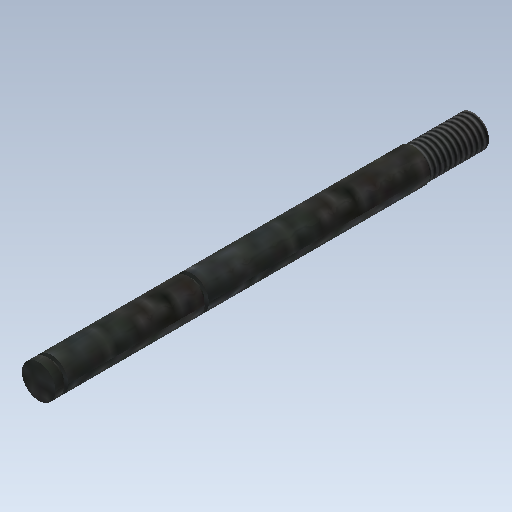
# Autodesk Inventor part: 500-104
Saved by Autodesk Inventor 2020 (Build 240168000, 168)
## iProperties
Created: 2015-04-18
Part Number: 500-104
Material: Steel
Document SubType Name: Modeling
Designer: Station9
Density: 7.85 g/cm^3
Appearance: Plate
Mass: 2.53931 g
Surface Area: 4.39374 cm^2
Volume: 0.323479 cm^3
Author: Station9
Autodesk Inventor part; units mm, degrees
ref_plane "YZ Plane" through (0, 0, 0) normal (1, 0, 0) x (0, 1, 0)
ref_plane "XZ Plane" through (0, 0, 0) normal (0, 1, 0) x (-1, 0, 0)
ref_plane "XY Plane" through (0, 0, 0) normal (0, 0, 1) x (1, 0, 0)
sketch "Sketch1" plane through (0, 0, 0) normal (0, 1, 0) x (-1, 0, 0)
  line L0 (0, 0) -> (1.6, 0)
  line L1 (1.6, -41.2616) -> (0, -41.2616)
  line L2 (0, -41.2616) -> (0, 0)
  line L3 (1.6, -0.8) -> (1.2, -0.8)
  line L4 (1.2, -0.8) -> (1.2, -1.2)
  line L5 (1.2, -1.2) -> (1.6, -1.2)
  line L6 (1.6, -14.1616) -> (1.2, -14.1616)
  line L7 (1.2, -14.1616) -> (1.2, -14.5616)
  line L8 (1.2, -14.5616) -> (1.6, -14.5616)
  line L9 (1.6, -35.5616) -> (1.5, -35.5616)
  line L10 (1.5, -35.5616) -> (1.5, -41.2616)
  line L11 (1.5, -41.2616) -> (1.6, -41.2616)
  line L12 (1.6, -14.5616) -> (1.6, -35.5616)
  line L13 (1.6, 0) -> (1.6, -0.8)
  line L14 (1.6, -1.2) -> (1.6, -14.1616)
  dimension "d0" = 5.7
  dimension "d1" = 21.4
  dimension "d2" = 0.8
  dimension "d3" = 0.4
  dimension "d4" = 1.2
  dimension "d6" = 0.4
  dimension "d7" = 1.5
  constraints: 30 end point, 7 parallel, 6 perpendicular, 4 horizontal, 2 point on line
  measures "d0" distance of L9.end L10.end
  measures "d1" distance between parallel lines of L9 L6
  measures "d2" distance from line of L3.end L0
  measures "d3" distance of L3.end L4.end
  measures "d4" distance between parallel lines of L2 L4
  measures "d6" distance of L6.end L7.end
  measures "d7" distance between parallel lines of L2 L10
revolve "Revolution1" add sketch "Sketch1" angle 360 about axis through (0, 0, -41.2616) along (0, 0, 1)
thread "Thread1" size "M3x0.5" class "6g" standard "ANSI Metric M Profile" full length
body "Solid1"
